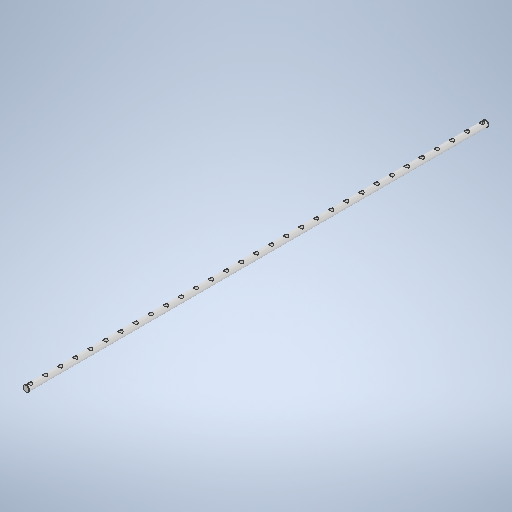
# Autodesk Inventor part: Tubo
Saved by Autodesk Inventor 2025.3 (Build 293356000, 356)
## iProperties
Created: 2025-11-02
Part Number: Tubo
Material: Genérico
Document SubType Name: Modeling
Designer: PAVILION
Density: 1 g/cm^3
Appearance: Valor por defecto
Author: PAVILION
Autodesk Inventor part; units mm, degrees
ref_plane "YZ Plane" through (0, 0, 0) normal (1, 0, 0) x (0, 1, 0)
ref_plane "XZ Plane" through (0, 0, 0) normal (0, 1, 0) x (-1, 0, 0)
ref_plane "XY Plane" through (0, 0, 0) normal (0, 0, 1) x (1, 0, 0)
sketch "Boceto1" plane through (0, 0, 0) normal (0, 0, 1) x (1, 0, 0)
  circle A0 centre (0, 0) radius 38.1
  circle A1 centre (0, 0) radius 34
  dimension "d0" = 76.2
  dimension "d1" = 68
  constraints: 2 centre point, 2 coincident
  measures "d0" diameter of A0
  measures "d1" diameter of A1
extrude "Extrusión1" add sketch "Boceto1" along normal blind 6100
sketch "Boceto2" plane through (0, 0, 6100) normal (0, 0, 1) x (1, 0, 0)
  circle A0 centre (0, 0) radius 39.5
  circle A1 centre (0, 0) radius 34 projected
  dimension "d4" = 79
  constraints: 1 centre point, 1 coincident
  measures "d4" diameter of A0
extrude "Extrusión2" add sketch "Boceto2" along normal blind 5 and the other way blind 5 contours A0 | A1
sketch "Boceto3" plane through (0, 0, 0) normal (0, 0, -1) x (-1, 0, 0)
  circle A0 centre (0, 0) radius 34 projected
  circle A1 centre (0, 0) radius 38.1 projected
  circle A2 centre (0, 0) radius 39.5 projected
extrude "Extrusión3" add sketch "Boceto3" along normal blind 5 and the other way blind 5 contours A0 | A1 | A2
sketch "Boceto4" plane through (0, 0, 0) normal (0, 1, 0) x (-1, 0, 0)
  line L0 (39.5, 6105) -> (-39.5, 6105) projected
  line L1 (39.5, 6105) -> (-39.5, 6105)
  line L2 (-39.5, 6105) -> (-39.5, -4.8433)
  line L3 (-39.5, -4.8433) -> (39.5, -4.8433)
  line L4 (39.5, -4.8433) -> (39.5, 6105)
  line L5 (0, 6105) -> (0, -4.8433)
  circle A0 centre (0, 3050.0783) radius 25
  circle A1 centre (0, 2850.0783) radius 25
  circle A2 centre (0, 3250.0783) radius 25
  circle A3 centre (0, 2650.0783) radius 25
  circle A4 centre (0, 3450.0783) radius 25
  circle A5 centre (0, 2450.0783) radius 25
  circle A6 centre (0, 3650.0783) radius 25
  circle A7 centre (0, 2250.0783) radius 25
  circle A8 centre (0, 3850.0783) radius 25
  circle A9 centre (0, 2050.0783) radius 25
  circle A10 centre (0, 4050.0783) radius 25
  circle A11 centre (0, 1850.0783) radius 25
  circle A12 centre (0, 4250.0783) radius 25
  circle A13 centre (0, 1650.0783) radius 25
  circle A14 centre (0, 4450.0783) radius 25
  circle A15 centre (0, 1450.0783) radius 25
  circle A16 centre (0, 4650.0783) radius 25
  circle A17 centre (0, 1250.0783) radius 25
  circle A18 centre (0, 4850.0783) radius 25
  circle A19 centre (0, 1050.0783) radius 25
  circle A20 centre (0, 5050.0783) radius 25
  circle A21 centre (0, 850.0783) radius 25
  circle A22 centre (0, 5250.0783) radius 25
  circle A23 centre (0, 650.0783) radius 25
  circle A24 centre (0, 5450.0783) radius 25
  circle A25 centre (0, 450.0783) radius 25
  circle A26 centre (0, 5650.0783) radius 25
  circle A27 centre (0, 250.0783) radius 25
  circle A28 centre (0, 5850.0783) radius 25
  circle A29 centre (0, 50.0783) radius 25
  circle A30 centre (0, 6050.0783) radius 25
  point P0 (0, 0)
  dimension "d13" = 50
  dimension "d16" = 200
  constraints: 31 centre point, 10 end point, 3 midpoint, 2 parallel, 1 horizontal, 1 perpendicular, 1 vertical, 60 other
  measures "d13" diameter of A0
  measures "d16" distance of A0.centre A1.centre
extrude "Extrusión4" cut sketch "Boceto4" along normal blind 50 contours A30 L5 | L5 A30 | A29 L5 | L5 A29 | A28 L5 | L5 A28 | A27 L5 | L5 A27 | A26 L5 | L5 A26 | A25 L5 | L5 A25 | A24 L5 | L5 A24 | A23 L5 | L5 A23 | A22 L5 | L5 A22 | A21 L5 | L5 A21 | A20 L5 | L5 A20 | A19 L5 | L5 A19 | A18 L5 | L5 A18 | A17 L5 | L5 A17 | A16 L5 | L5 A16 | A15 L5 | L5 A15 | A14 L5 | L5 A14 | A13 L5 | L5 A13 | A12 L5 | L5 A12 | A11 L5 | L5 A11 | A10 L5 | L5 A10 | A9 L5 | L5 A9 | A8 L5 | L5 A8 | A7 L5 | L5 A7 | A6 L5 | L5 A6 | A5 L5 | L5 A5 | A4 L5 | L5 A4 | A3 L5 | L5 A3 | A2 L5 | L5 A2 | A1 L5 | L5 A1 | A0 L5 | L5 A0
equation "\"d21\" = d13"
